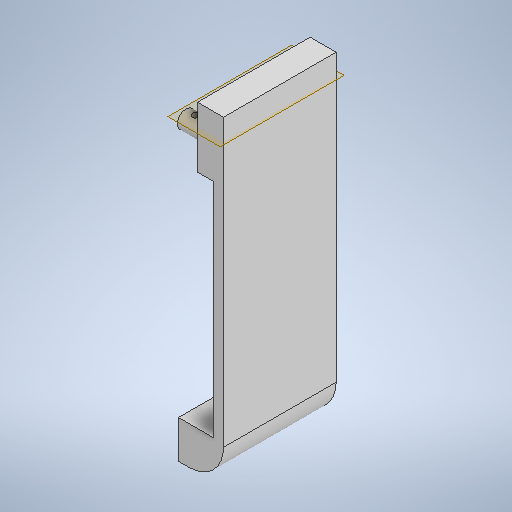
# Autodesk Inventor part: hook_applicator_slide in
Saved by Autodesk Inventor 2026.1 (Build 301233020, 233B)
## iProperties
Created: 2025-12-05
Part Number: hook_applicator_slide in
Material: Generisch
Document SubType Name: Modeling
Designer: sarae
Density: 1 g/cm^3
Appearance: Vorgabe
Author: sarae
Autodesk Inventor part; units mm, degrees
ref_plane "YZ Plane" through (0, 0, 0) normal (1, 0, 0) x (0, 1, 0)
ref_plane "XZ Plane" through (0, 0, 0) normal (0, 1, 0) x (-1, 0, 0)
ref_plane "XY Plane" through (0, 0, 0) normal (0, 0, 1) x (1, 0, 0)
sketch "Skizze1" plane through (0, 0, 0) normal (0, 1, 0) x (-1, 0, 0)
  line L0 (1.2301, 16.646) -> (-1.7699, 16.646)
  line L1 (-1.7699, 16.646) -> (-1.7699, 9.646)
  line L2 (-1.7699, 9.646) -> (1.2301, 9.646)
  line L3 (1.2301, 9.646) -> (1.2301, 16.646)
  line L4 (-1.7699, 9.646) -> (-0.5699, 9.646)
  line L5 (-0.5699, 9.646) -> (-0.5699, -20.354)
  line L6 (-0.5699, -20.354) -> (-1.7699, -20.354)
  line L7 (-1.7699, -20.354) -> (-1.7699, 9.646)
  line L8 (-0.5699, -20.354) -> (3.4301, -20.354)
  line L9 (3.4301, -20.354) -> (3.4301, -15.9771)
  line L10 (3.4301, -15.9771) -> (-0.5699, -15.9771)
  line L11 (-0.5699, -15.9771) -> (-0.5699, -20.354)
  point P0 (0, 0)
  dimension "d0" = 3
  dimension "d1" = 7
  dimension "d2" = 1.2
  dimension "d3" = 30
  dimension "d4" = 4
  constraints: 24 end point, 6 parallel, 3 horizontal, 3 perpendicular
  measures "d0" distance of L2.end L1.end
  measures "d1" distance of L1.end L0.end
  measures "d2" distance of L5.end L6.end
  measures "d3" distance of L4.end L5.end
  measures "d4" distance of L10.end L9.end
extrude "Extrusion1" add sketch "Skizze1" along normal blind 13
fillet "Rundung1" radius 4 1 edges at (1.7699, 6.5, -20.354)
sketch "Skizze2" plane through (0, 13, 0) normal (0, 1, 0) x (1, 0, 0)
  line L0 (0.5699, -9.646) -> (-1.2301, -9.646) projected
  line L1 (0.5699, -9.646) -> (-0.1301, -9.646)
  line L2 (-0.1301, -9.646) -> (-0.1301, -14.642)
  line L3 (-0.1301, -14.642) -> (0.5699, -14.642)
  line L4 (0.5699, -14.642) -> (0.5699, -9.646)
  point P0 (0, 0)
  point P1 (-0.3301, -9.646)
  point P2 (-0.1301, -9.646)
  dimension "d8" = 5
  dimension "d9" = 0.7
  constraints: 8 end point, 2 parallel, 1 horizontal, 1 midpoint, 1 perpendicular
  measures "d8" distance of L2.end point (-0.33, -9.646)
  measures "d9" distance between parallel lines of L2 L4
sketch "Skizze3" plane through (0, 13, 0) normal (0, 1, 0) x (1, 0, 0)
  line L0 (-3.4301, 20.354) -> (-3.4301, 15.9771) projected
  line L1 (-3.4301, 15.9771) -> (0.5699, 15.9771) projected
  arc A0 (0.5699, 15.9771) -> (-2.5715, 19.8839) centre (-3.4301, 15.9771) ccw
  line L2 (0.5699, 15.9771) -> (0.5699, -9.646) projected
  line L3 (0.5699, 15.9771) -> (-0.0301, 15.9771)
  arc A1 (-0.0301, 15.9771) -> (-2.8554, 19.3282) centre (-3.4301, 15.9771) ccw
  line L4 (-2.8554, 19.3282) -> (-2.5715, 19.8839)
  point P0 (0, 0)
  dimension "d10" = 0.6
  constraints: 4 end point, 4 point on circle, 2 centre point, 1 coincident, 1 point on line
  measures "d10" distance of L1.end L3.end
extrude "Extrusion2" cut sketch "Skizze3" against normal blind 12
extrude "Extrusion3" cut sketch "Skizze2" against normal blind 12
sketch "Skizze4" plane through (-1.2301, 0, 9.646) normal (-1, 0, 0) x (0, 0, 1)
  line L0 (0, 0) -> (7, 0) projected
  line L1 (7, 0) -> (3.5, 0)
  line L2 (4.996, 13) -> (0, 13) projected
  line L3 (3.5, 13) -> (3.5, 0)
  line L4 (3.5, 6.5) -> (7, 6.5)
  line L5 (7, 0) -> (7, 13) projected
  circle A0 centre (3.5, 6.5) radius 1
  circle A1 centre (3.5, 1.1664) radius 1
  circle A2 centre (3.5, 3.7221) radius 1
  circle A3 centre (3.5, 8.9382) radius 1
  circle A4 centre (3.5, 11.2973) radius 1
  point P0 (-9.646, 0)
  dimension "d15" = 2
  dimension "d16" = 2
  dimension "d17" = 2
  dimension "d18" = 2
  dimension "d19" = 2
  constraints: 6 end point, 5 centre point, 5 point on line, 3 midpoint, 1 coincident, 1 perpendicular
  measures "d15" diameter of A0
  measures "d16" diameter of A1
  measures "d17" diameter of A2
  measures "d18" diameter of A3
  measures "d19" diameter of A4
extrude "Extrusion4" add sketch "Skizze4" along normal blind 2.5 contours A4 L3 | L3 A4 | A3 L3 | L3 A3 | A1 L3 | L3 A1 | A0 L3 L4 | L4 L3 A0 | A2 L3 | L3 A2 | L3 A0
ref_plane "Arbeitsebene1" through (-1.2301, 11.2973, 14.146) normal (0, 0, 1) x (1, 0, 0)
sketch "Skizze5" plane through (-1.2301, 11.2973, 14.146) normal (0, 0, 1) x (1, 0, 0)
  line L0 (-2.2, -11.2973) -> (-2.2, 1.7027) projected
  ellipse E0 centre (-0.7, -4.7973) end of major axis (-0.7, -3.6152) minor radius 0.3015
  ellipse E1 centre (-0.7, -2.3523) end of major axis (-0.7, -1.125) minor radius 0.2616
  line L1 (0, -1.3591) -> (-2.5, -1.3591) projected
  ellipse E2 centre (-0.7, 0.0155) end of major axis (-0.7, 1.1416) minor radius 0.2973
  circle A0 centre (-1.25, -10.1312) radius 0.3762
  ellipse E3 centre (-0.7, -7.4834) end of major axis (-0.7, -8.7492) minor radius 0.3
  line L2 (0, -8.5752) -> (-2.5, -8.5752) projected
  point P0 (1.2301, -11.2973)
  point P1 (-0.8518, -8.5752)
  point P2 (-0.5482, -8.5752)
  constraints: 2 horizontal, 1 centre point, 8 other
extrude "Extrusion5" cut sketch "Skizze5" against normal blind 1 contours E1 L1 | L1 E1 | E3 L2 | E0 | E2 picked at (-0.7898, -7.5169)
sketch "Skizze6" plane through (-1.2301, 11.2973, 14.146) normal (0, 0, 1) x (1, 0, 0)
  circle A0 centre (-1.315, -10.1413) radius 0.3946
  point P0 (1.2301, -11.2973)
  constraints: 1 centre point
extrude "Extrusion6" cut sketch "Skizze6" against normal blind 2.5
